makerbeam-arcade-button-mount v2 (Autodesk Fusion 360 design; units mm, degrees)
Autodesk Fusion 360 part; units mm, degrees
box "BoxPrimitive1" add length 60 width 60 height 2 placed x (0, 0, -1) y (-1, 0, 0) z (0, 1, 0) at (60, 0, 0) makes body 1
box "BoxPrimitive2" add length 60 width 2 height 10 placed x (0, 0, -1) y (-1, 0, 0) z (0, 1, 0) at (2, 0, 0) bodies 1
box "BoxPrimitive3" add length 60 width 2 height 10 placed x (0, 0, -1) y (-1, 0, 0) z (0, 1, 0) at (60, 0, 0) bodies 1
cylinder "CylinderPrimitive1" cut diameter 3 height -70 placed x (0, 0, -1) y (0, 1, 0) z (1, 0, 0) at (60, 5, -5) bodies 1
cylinder "CylinderPrimitive2" cut diameter 3 height -75 placed x (0, 0, -1) y (0, 1, 0) z (1, 0, 0) at (60, 5, -55) bodies 1
cylinder "CylinderPrimitive3" cut diameter 30 height -30 placed x (1, 0, 0) y (0, 0, -1) z (0, 1, 0) at (30, 2, -30) bodies 1
box "BoxPrimitive4" cut length 8 width 4 height -8 placed x (0, 0, -1) y (-1, 0, 0) z (0, 1, 0) at (32, 2, -50) bodies 1
box "BoxPrimitive5" cut length 8 width 4 height -9 placed x (0, 0, -1) y (-1, 0, 0) z (0, 1, 0) at (32, 2, -2) bodies 1
box "BoxPrimitive6" cut length 10 width 13 height -10 placed x (0, 0, -1) y (-1, 0, 0) z (0, 1, 0) at (58, 2, -50) bodies 1
box "BoxPrimitive7" cut length 10 width 13 height -10 placed x (0, 0, 1) y (1, 0, 0) z (0, 1, 0) at (2, 2, -60) bodies 1
box "BoxPrimitive8" cut length 10 width 13 height -10 placed x (0, 0, 1) y (1, 0, 0) z (0, 1, 0) at (45, 2, -10) bodies 1
box "BoxPrimitive9" cut length 10 width 13 height -10 placed x (0, 0, -1) y (-1, 0, 0) z (0, 1, 0) at (15, 2, 0) bodies 1
sketch "Sketch13" plane through (0, 0, 0) normal (0, 0, 1) x (1, 0, 0)
  line L0 (58, 2) -> (45, 2)
  line L1 (58, 2) -> (58, 10)
  line L2 (45, 2) -> (58, 2)
  line L3 (58, 10) -> (50, 2)
  point P0 (58, 2)
  point P1 (58, 10)
extrude "Extrude1" add sketch "Sketch13" along normal blind 2 separate body makes body 2
move_body "Move1" bodies 2 to x (1, 0, 0) y (0, 1, 0) z (0, 0, 1) at (0, 0, -12)
copy_body "CopyPasteBodies1" bodies 2 makes body 3
move_body "Move2" bodies 3 to x (1, 0, 0) y (0, 1, 0) z (0, 0, 1) at (0, 0, -38)
sketch "Sketch14" plane through (0, 0, 0) normal (0, 0, 1) x (1, 0, 0)
  line L0 (2, 2) -> (15, 2)
  line L1 (15, 2) -> (2, 2)
  line L2 (2, 10) -> (10, 2)
  line L3 (2, 2) -> (2, 10)
  point P0 (2, 10)
extrude "Extrude2" add sketch "Sketch14" along normal blind 2 separate body makes body 4
move_body "Move3" bodies 4 to x (1, 0, 0) y (0, 1, 0) z (0, 0, 1) at (0, 0, -12)
copy_body "CopyPasteBodies2" bodies 4 makes body 5
move_body "Move4" bodies 5 to x (1, 0, 0) y (0, 1, 0) z (0, 0, 1) at (0, 0, -38)
